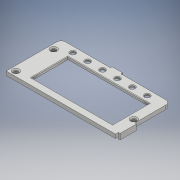
# Autodesk Inventor part: front
Saved by Autodesk Inventor 2017 (Build 210142000, 142)
## iProperties
Created: 2017-07-31
Part Number: front
Material: Generic
Document SubType Name: Modeling
Designer: Käyttäjä
Density: 1 g/cm^3
Appearance: Default
Author: Käyttäjä
Autodesk Inventor part; units mm, degrees
ref_plane "YZ Plane" through (0, 0, 0) normal (1, 0, 0) x (0, 1, 0)
ref_plane "XZ Plane" through (0, 0, 0) normal (0, 1, 0) x (-1, 0, 0)
ref_plane "XY Plane" through (0, 0, 0) normal (0, 0, 1) x (1, 0, 0)
sketch "Sketch1" plane through (0, 0, 0) normal (0, 0, 1) x (1, 0, 0)
  line L0 (0, 0) -> (95.5, 0)
  line L1 (95.5, 0) -> (95.5, 44)
  line L2 (91.5, 48) -> (4, 48)
  line L3 (0, 44) -> (0, 0)
  arc A0 (4, 48) -> (0, 44) centre (4, 44) ccw
  arc A1 (95.5, 44) -> (91.5, 48) centre (91.5, 44) ccw
  line L4 (0, -38) -> (95.5, -38) construction
  line L5 (16, 38) -> (87, 38)
  line L6 (87, 38) -> (87, 6)
  line L7 (87, 6) -> (16, 6)
  line L8 (16, 6) -> (16, 38)
  circle A2 centre (15.25, 43) radius 2
  circle A3 centre (28.25, 43) radius 2
  circle A4 centre (41.25, 43) radius 2
  circle A5 centre (54.25, 43) radius 2
  circle A6 centre (67.25, 43) radius 2
  circle A7 centre (80.25, 43) radius 2
  point P0 (95.5, 48)
  point P1 (0, 48)
  dimension "d0" = 95.5
  dimension "d1" = 48
  dimension "d2" = 4
  dimension "d3" = 86
  dimension "d6" = 16
  dimension "d8" = 8.5
  dimension "d9" = 15.25
  dimension "d14" = 13
  dimension "d19" = 4
  dimension "d20" = 81
  dimension "d66" = 10
  dimension "d67" = 6
  constraints: 18 end point, 8 centre point, 4 horizontal, 4 parallel, 4 point on circle, 4 point on line, 4 tangent, 2 perpendicular, 1 equal radius, 10 other
  measures "d0" distance of point (95.5, 48) point (0, 48)
  measures "d1" distance of point (0, 48) L0.start
  measures "d2" radius of A0
  measures "d3" distance between parallel lines of L4 L2
  measures "d6" distance between parallel lines of L3 L8
  measures "d8" distance between parallel lines of L1 L6
  measures "d9" distance from line of L3 A2.centre
  measures "d14" distance of A2.centre A3.centre
  measures "d19" diameter of A2
  measures "d20" distance from line of A2.centre L4
  measures "d66" distance between parallel lines of L2 L5
  measures "d67" distance between parallel lines of L0 L7
extrude "Extrusion1" add sketch "Sketch1" along normal blind 1.4
sketch "Sketch2" plane through (0, 0, 0) normal (0, 0, -1) x (-1, 0, 0)
  line L0 (-87, 6) -> (-87, 38) projected
  line L1 (-87, 38) -> (-16, 38) projected
  line L2 (-16, 38) -> (-16, 6) projected
  line L3 (-16, 6) -> (-87, 6) projected
  circle A0 centre (-80.25, 43) radius 2 projected
  circle A1 centre (-67.25, 43) radius 2 projected
  circle A2 centre (-54.25, 43) radius 2 projected
  circle A3 centre (-41.25, 43) radius 2 projected
  circle A4 centre (-28.25, 43) radius 2 projected
  circle A5 centre (-15.25, 43) radius 2 projected
  line L4 (0, 0) -> (-95.5, 0) projected
  line L5 (0, 44) -> (0, 0) projected
  arc A6 (0, 44) -> (-4, 48) centre (-4, 44) ccw projected
  line L6 (-91.5, 48) -> (-4, 48) projected
  arc A7 (-91.5, 48) -> (-95.5, 44) centre (-91.5, 44) ccw projected
  line L7 (-95.5, 0) -> (-95.5, 44) projected
  line L8 (-1, 1) -> (-94.5, 1)
  line L9 (-94.5, 1) -> (-94.5, 46.6458)
  line L10 (-87, 47) -> (-16, 47)
  line L11 (-1, 46.6458) -> (-1, 1)
  line L12 (0, 0) -> (-95.5, 0) projected
  line L13 (-16, 47) -> (-16, 48)
  line L14 (-91.5, 48) -> (-4, 48) projected
  line L15 (-87, 47) -> (-87, 48)
  point P0 (-94.5, 44)
  point P1 (-1, 44)
  dimension "d23" = 1
  dimension "d26" = 1
  dimension "d27" = 1
  dimension "d28" = 1
  constraints: 12 end point, 4 point on line, 2 point on circle, 2 vertical alignment, 1 parallel, 1 vertical
  measures "d23" distance between parallel lines of L5 L11
  measures "d26" distance between parallel lines of L7 L9
  measures "d27" distance between parallel lines of L6 L10
  measures "d28" distance between parallel lines of L4 L8
extrude "edge" add sketch "Sketch2" along normal blind 2 contours L4 L7 A7 L9 L8 L11 A6 L5
sketch "Sketch3" plane through (0, 0, 1.4) normal (0, 0, 1) x (1, 0, 0)
  circle A0 centre (4.25, 37.25) radius 1.75
  circle A1 centre (4.25, 4.25) radius 1.75
  circle A2 centre (92.25, 19.25) radius 1.75
  line L0 (91.5, 48) -> (4, 48) projected
  line L1 (0, 44) -> (0, 0) projected
  line L2 (95.5, 0) -> (95.5, 44) projected
  line L3 (0, 0) -> (95.5, 0) projected
  dimension "d29" = 3.5
  dimension "d30" = 33
  dimension "d31" = 10.75
  dimension "d32" = 4.25
  dimension "d33" = 3.25
  dimension "d35" = 28.75
  constraints: 3 centre point, 2 equal radius, 1 vertical alignment
  measures "d29" diameter of A0
  measures "d30" distance of A1.centre A0.centre
  measures "d31" distance from line of A0.centre L0
  measures "d32" distance from line of L1 A0.centre
  measures "d33" distance from line of A2.centre L2
  measures "d35" distance from line of L0 A2.centre
extrude "Extrusion3" cut sketch "Sketch3" against normal blind 1.5
sketch "Sketch4" plane through (0, 0, 0) normal (0, 0, -1) x (-1, 0, 0)
  circle A0 centre (-4.25, 4.25) radius 1.75 projected
  circle A1 centre (-4.25, 37.25) radius 1.75 projected
  circle A2 centre (-92.25, 19.25) radius 1.75 projected
  line L0 (-1, 1) -> (-1, 46.6458) projected
  arc A3 (-1, 46.6458) -> (-4, 48) centre (-4, 44) ccw projected
  line L1 (-91.5, 48) -> (-4, 48) projected
  arc A4 (-91.5, 48) -> (-94.5, 46.6458) centre (-91.5, 44) ccw projected
  line L2 (-94.5, 46.6458) -> (-94.5, 1) projected
  line L3 (-94.5, 1) -> (-1, 1) projected
  line L4 (-87, 6) -> (-87, 38) projected
  line L5 (-87, 38) -> (-16, 38) projected
  line L6 (-16, 38) -> (-16, 6) projected
  line L7 (-16, 6) -> (-87, 6) projected
  circle A5 centre (-80.25, 43) radius 2 projected
  circle A6 centre (-67.25, 43) radius 2 projected
  circle A7 centre (-54.25, 43) radius 2 projected
  circle A8 centre (-41.25, 43) radius 2 projected
  circle A9 centre (-28.25, 43) radius 2 projected
  circle A10 centre (-15.25, 43) radius 2 projected
  arc A11 (-7, 2.0849) -> (-7, 6.4151) centre (-4.25, 4.25) ccw
  arc A12 (-7, 35.0849) -> (-7, 39.4151) centre (-4.25, 37.25) ccw
  line L8 (-7, 2.0849) -> (-7, 6.4151)
  line L9 (-7, 35.0849) -> (-7, 39.4151)
  line L10 (-89, 17.951) -> (-89, 20.549)
  arc A13 (-94.5, 16.569) -> (-89, 17.951) centre (-92.25, 19.25) ccw
  arc A14 (-89, 20.549) -> (-94.5, 21.931) centre (-92.25, 19.25) ccw
  point P0 (0, 0)
  dimension "d38" = 7
  dimension "d39" = 7
  dimension "d41" = 1.5
  dimension "d42" = 2
  dimension "d43" = 3.5
  constraints: 8 point on circle, 6 end point, 4 centre point, 4 point on line, 3 coincident, 2 vertical, 1 concentric
  measures "d38" diameter of A11
  measures "d39" diameter of A12
  measures "d42" distance between parallel lines of L4 L10
  measures "d43" radius of A13
extrude "Extrusion4" add sketch "Sketch4" along normal blind 2 contours A11 L3 L8 L0 | L0 A11 | A11 L3 | A12 L9 L0 | L0 A12 | L2 A14 L10 A13
sketch "Sketch5" plane through (0, 0, 0) normal (0, 0, -1) x (-1, 0, 0)
  line L0 (-46.25, 48) -> (-49.25, 48)
  line L1 (-49.25, 48) -> (-49.25, 47)
  line L2 (-49.25, 47) -> (-46.25, 47)
  line L3 (-46.25, 47) -> (-46.25, 48)
  line L4 (-16, 6) -> (-87, 6) projected
  line L5 (-91.5, 48) -> (-4, 48) projected
  point P0 (0, 0)
  point P1 (-51.5, 6)
  point P2 (-47.75, 48)
  point P3 (-47.75, 47)
  dimension "d44" = 1
  dimension "d45" = 3
  constraints: 8 end point, 3 midpoint, 2 parallel, 1 horizontal, 1 perpendicular, 1 point on line, 1 vertical alignment
  measures "d44" distance of L2.end L0.start
  measures "d45" distance of L1.end L2.end
extrude "Extrusion5" add sketch "Sketch5" along normal blind 2
chamfer "Chamfer1" distance 1.2 angle 45 3 edges at (2.5, 37.25, 1.4) (2.5, 4.25, 1.4) (90.5, 19.25, 1.4)
fillet "Fillet1" radius 0.5 10 edges at (13.25, 43, 1.4) (26.25, 43, 1.4) (39.25, 43, 1.4) (52.25, 43, 1.4) (65.25, 43, 1.4) (78.25, 43, 1.4) (51.5, 38, 1.4) (87, 22, 1.4) (51.5, 6, 1.4) (16, 22, 1.4)
fillet "Fillet2" radius 1 3 edges at (2.5, 4.25, 0.2) (2.5, 37.25, 0.2) (90.5, 19.25, 0.2)
sketch "Sketch6" plane through (0, 0, 1.4) normal (0, 0, 1) x (1, 0, 0)
  line L0 (91.5, 48) -> (4, 48) projected
  line L1 (43, 48) -> (52.5, 48)
  line L2 (52.5, 48) -> (52.5, 49.5)
  line L3 (52.5, 49.5) -> (43, 49.5)
  line L4 (43, 49.5) -> (43, 48)
  line L5 (95.5, 0) -> (95.5, 44) projected
  line L6 (95.5, 17) -> (97, 17)
  line L7 (97, 17) -> (97, 2.5)
  line L8 (97, 2.5) -> (95.5, 2.5)
  line L9 (95.5, 2.5) -> (95.5, 17)
  point P0 (0, 0)
  point P1 (47.75, 49.5)
  point P2 (47.75, 48)
  dimension "d55" = 1.5
  dimension "d56" = 9.5
  dimension "d57" = 1.5
  dimension "d58" = 31
  dimension "d59" = 14.5
  constraints: 16 end point, 4 parallel, 2 horizontal, 2 midpoint, 2 perpendicular, 2 point on line, 1 vertical alignment
  measures "d55" distance of L3.end L1.start
  measures "d56" distance of L2.end L3.end
  measures "d57" distance of L6.start L6.end
  measures "d58" distance between parallel lines of L0 L6
  measures "d59" distance of L6.end L7.end
extrude "Extrusion6" add sketch "Sketch6" against normal blind 5
sketch "Sketch7" plane through (0, 0, 0) normal (0, 0, -1) x (-1, 0, 0)
  line L0 (-49.25, 47) -> (-49.25, 48) projected
  line L1 (-91.5, 48) -> (-52.5, 48) projected
  arc A0 (-91.5, 48) -> (-94.5, 46.6458) centre (-91.5, 44) ccw projected
  line L2 (-94.5, 46.6458) -> (-94.5, 21.931) projected
  arc A1 (-89, 20.549) -> (-94.5, 21.931) centre (-92.25, 19.25) ccw projected
  line L3 (-89, 20.549) -> (-89, 17.951) projected
  arc A2 (-94.5, 16.569) -> (-89, 17.951) centre (-92.25, 19.25) ccw projected
  line L4 (-94.5, 16.569) -> (-94.5, 1) projected
  line L5 (-94.5, 1) -> (-5.549, 1) projected
  arc A3 (-7, 2.0849) -> (-5.549, 1) centre (-4.25, 4.25) ccw projected
  line L6 (-7, 2.0849) -> (-7, 6.4151) projected
  arc A4 (-1, 5.549) -> (-7, 6.4151) centre (-4.25, 4.25) ccw projected
  line L7 (-1, 5.549) -> (-1, 35.951) projected
  arc A5 (-7, 35.0849) -> (-1, 35.951) centre (-4.25, 37.25) ccw projected
  line L8 (-7, 35.0849) -> (-7, 39.4151) projected
  arc A6 (-1, 38.549) -> (-7, 39.4151) centre (-4.25, 37.25) ccw projected
  line L9 (-1, 38.549) -> (-1, 46.6458) projected
  arc A7 (-1, 46.6458) -> (-4, 48) centre (-4, 44) ccw projected
  line L10 (-43, 48) -> (-4, 48) projected
  line L11 (-46.25, 48) -> (-43, 48) projected
  line L12 (-46.25, 48) -> (-46.25, 47) projected
  line L13 (-46.25, 47) -> (-49.25, 47) projected
  circle A8 centre (-15.25, 43) radius 2 projected
  circle A9 centre (-28.25, 43) radius 2 projected
  circle A10 centre (-41.25, 43) radius 2 projected
  circle A11 centre (-54.25, 43) radius 2 projected
  circle A12 centre (-67.25, 43) radius 2 projected
  circle A13 centre (-80.25, 43) radius 2 projected
  line L14 (-87, 6) -> (-87, 38) projected
  line L15 (-87, 38) -> (-16, 38) projected
  line L16 (-16, 38) -> (-16, 6) projected
  line L17 (-16, 6) -> (-87, 6) projected
  line L18 (-15, 5) -> (-15, 39)
  line L19 (-15, 39) -> (-88, 39)
  line L20 (-88, 39) -> (-88, 5)
  line L21 (-88, 5) -> (-15, 5)
  line L22 (-52.5, 48) -> (-49.25, 48) projected
  point P0 (0, 0)
  dimension "d63" = 1
  constraints: 8 end point, 3 other
  measures "d63" distance between parallel lines of L16 L18
extrude "Extrusion7" add sketch "Sketch7" along normal blind 1 contours L21 L20 L19 L18
body "Solid1"
